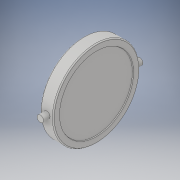
# Autodesk Inventor part: Espejo
Saved by Autodesk Inventor 2018 (Build 220112000, 112)
## iProperties
Created: 2018-05-29
Part Number: Espejo
Material: Generic
Document SubType Name: Modeling
Designer: dm0814
Density: 1 g/cm^3
Appearance: Default
Author: dm0814
Autodesk Inventor part; units mm, degrees
ref_plane "YZ Plane" through (0, 0, 0) normal (1, 0, 0) x (0, 1, 0)
ref_plane "XY Plane" through (0, 0, 0) normal (0, 0, 1) x (1, 0, 0)
sketch "Sketch1" plane through (0, 0, 0) normal (0, 1, 0) x (-1, 0, 0)
  line L0 (0, 11.35) -> (0, 12.95)
  line L1 (0.3, 13.25) -> (3.7, 13.25)
  line L2 (0, -11.35) -> (0, -13.25)
  line L3 (0, -13.25) -> (4, -13.25)
  line L4 (4, 12.95) -> (4, 11.25)
  line L5 (4, -13.25) -> (4, -11.25)
  arc A0 (4, 11.25) -> (4, -11.25) centre (34.6406, 0) ccw
  line L6 (0.25, 11.25) -> (0.25, 11.25)
  line L7 (0.25, 11.25) -> (0.25, -11.25)
  line L8 (0.25, -11.25) -> (0.25, -11.25)
  arc A1 (4, 12.95) -> (3.7, 13.25) centre (3.7, 12.95) ccw
  arc A2 (0.3, 13.25) -> (0, 12.95) centre (0.3, 12.95) ccw
  line L9 (0, 11.35) -> (0.25, 11.25)
  line L10 (0, -11.35) -> (0.25, -11.25)
  line L11 (0, 0) -> (3.4534, 0)
  line L12 (2, 0) -> (0.25, 0)
  point P0 (0, 13.25)
  point P1 (4, 13.25)
  point P2 (0, 11.25)
  point P3 (0, -11.25)
  dimension "d0" = 13.25
  dimension "d1" = 26.5
  dimension "d2" = 4
  dimension "d4" = 2
  dimension "d5" = 2
  dimension "d6" = 0.25
  dimension "d7" = 0.3
  dimension "d8" = 0.1
  dimension "d9" = 0.25
  dimension "d10" = 0.1
  dimension "d11" = 0.25
  constraints: 26 end point, 11 point on line, 7 point on circle, 4 perpendicular, 4 tangent, 3 centre point, 3 vertical, 1 equal radius, 1 horizontal, 1 midpoint, 1 parallel
  measures "d0" distance of L11.start point (0, 13.25)
  measures "d1" distance of point (4, 13.25) L3.end
  measures "d2" distance of point (0, 13.25) point (4, 13.25)
  measures "d4" distance of point (4, 13.25) L4.end
  measures "d5" distance of L3.end L5.end
  measures "d6" distance of point (0, 11.25) L6.end
  measures "d7" radius of A1
  measures "d8" distance of L0.start point (0, 11.25)
  measures "d9" distance of L6.start point (0, 11.25)
  measures "d10" distance of L2.start point (0, -11.25)
  measures "d11" distance of L8.end point (0, -11.25)
revolve "Revolution1" add sketch "Sketch1" angle 360 about axis through (0, 0, 0) along (-1, 0, 0) contours L0 A2 L1 A1 L4 A0 L11 L7 L9
ref_plane "Work Plane1" through (-2, 13.25, 0) normal (0, 1, 0) x (-1, 0, 0)
sketch "Sketch2" plane through (-2, 13.25, 0) normal (0, 1, 0) x (-1, 0, 0)
  arc A0 (2, 11.25) -> (2, -11.25) centre (32.6406, 0) ccw projected
  circle A1 centre (0, 0) radius 1
  point P0 (-2, 0)
  dimension "d13" = 2
  constraints: 1 centre point, 1 point on circle
  measures "d13" diameter of A1
extrude "Extrusion1" add sketch "Sketch2" along normal blind 2 and the other way blind 1
pattern_circular "Circular Pattern1" count 2 over 360 about axis through (-2, 0, 0) along (-1, 0, 0) of "Extrusion1"
ref_plane "Work Plane2" through (-2, -13.25, 0) normal (0, -1, 0) x (-1, 0, 0)
equation "\"d10\" = d8"
equation "\"d11\" = d9"
body "Solid1"
